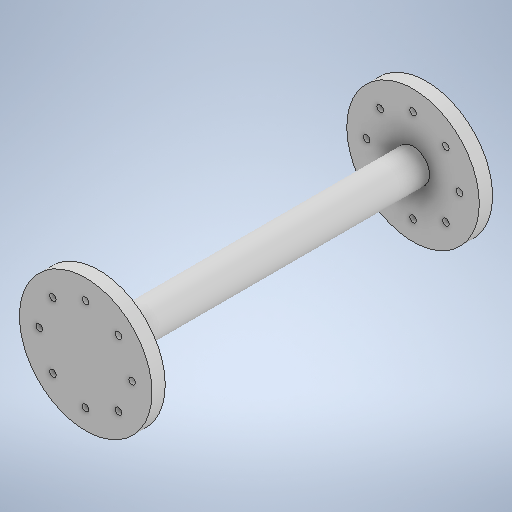
# Autodesk Inventor part: サーボパーツ2
Saved by Autodesk Inventor 2025.1 (Build 291241000, 241)
## iProperties
Created: 2026-05-20
Part Number: サーボパーツ2
Material: 一般
Document SubType Name: Modeling
Designer: takan
Density: 1 g/cm^3
Appearance: 既定
Author: takan
Autodesk Inventor part; units mm, degrees
ref_plane "YZ Plane" through (0, 0, 0) normal (1, 0, 0) x (0, 1, 0)
ref_plane "XZ Plane" through (0, 0, 0) normal (0, 1, 0) x (-1, 0, 0)
ref_plane "XY Plane" through (0, 0, 0) normal (0, 0, 1) x (1, 0, 0)
sketch "スケッチ1" plane through (0, 0, 0) normal (0, 0, 1) x (1, 0, 0)
  circle A0 centre (0, 0) radius 2.5
  dimension "d0" = 5
  constraints: 1 centre point, 1 coincident
  measures "d0" diameter of A0
extrude "押し出し1" add sketch "スケッチ1" along normal mid plane 51.4
sketch "スケッチ2" plane through (0, 0, 25.7) normal (0, 0, 1) x (1, 0, 0)
  circle A0 centre (0, 0) radius 10
  dimension "d3" = 20
  constraints: 1 centre point, 1 coincident
  measures "d3" diameter of A0
extrude "押し出し2" add sketch "スケッチ2" against normal blind 2
sketch "スケッチ3" plane through (0, 0, -25.7) normal (0, 0, -1) x (-1, 0, 0)
  circle A0 centre (0, 0) radius 10
  dimension "d6" = 20
  constraints: 1 centre point, 1 coincident
  measures "d6" diameter of A0
extrude "押し出し3" add sketch "スケッチ3" against normal blind 2
sketch "スケッチ4" plane through (0, 0, -25.7) normal (0, 0, -1) x (-1, 0, 0)
  point P0 (0, 0)
  point P1 (7, 0)
  point P2 (4.9497, 4.9497)
  point P3 (0, 7)
  point P4 (-4.9497, 4.9497)
  point P5 (-7, 0)
  point P6 (-4.9497, -4.9497)
  point P7 (0, -7)
  point P8 (4.9497, -4.9497)
  dimension "d9" = 7
  dimension "d12" = 360
  constraints: 9 other
  measures "d9" distance of point (0, 0) point (7, 0)
hole "穴1" at (-7, 0, -25.7) at (-4.9497, 4.9497, -25.7) at (0, 7, -25.7) at (4.9497, 4.9497, -25.7) at (7, 0, -25.7) at (4.9497, -4.9497, -25.7) at (0, -7, -25.7) at (-4.9497, -4.9497, -25.7) direction (0, 0, 1) diameter 1 end through all
